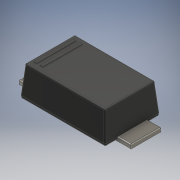
# Autodesk Inventor part: Semiconductor_DO219AB
Saved by Autodesk Inventor 2018 (Build 220112000, 112)
## iProperties
Created: 2018-09-29
Part Number: Semiconductor_DO219AB
Material: ABS Plastic
Document SubType Name: Modeling
Designer: Bradley
Density: 1.06 g/cm^3
Appearance: Smooth - Black
Author: Bradley
Autodesk Inventor part; units mm, degrees
ref_plane "YZ Plane" through (0, 0, 0) normal (1, 0, 0) x (0, 1, 0)
ref_plane "XZ Plane" through (0, 0, 0) normal (0, 1, 0) x (-1, 0, 0)
ref_plane "XY Plane" through (0, 0, 0) normal (0, 0, 1) x (1, 0, 0)
sketch "Sketch1" plane through (0, 0, 0) normal (0, 0, 1) x (1, 0, 0)
  line L0 (-1.4, -0.9) -> (1.4, -0.9)
  line L1 (1.4, -0.9) -> (1.4, 0.9)
  line L2 (1.4, 0.9) -> (-1.4, 0.9)
  line L3 (-1.4, 0.9) -> (-1.4, -0.9)
  line L4 (-1.4, -0.9) -> (1.4, 0.9) construction
  line L5 (1.4, -0.9) -> (-1.4, 0.9) construction
  point P0 (0, 0)
  dimension "d0" = 2.8
  dimension "d1" = 1.8
  constraints: 12 end point, 2 midpoint, 2 parallel, 1 horizontal, 1 perpendicular
  measures "d0" distance of L2.end L1.end
  measures "d1" distance of L1.end L0.end
extrude "Extrusion1" add sketch "Sketch1" along normal blind 0.9 draft -5 and the other way blind 0.1 draft -5
sketch "Sketch2" plane through (0, 0, 0) normal (0, 0, 1) x (1, 0, 0)
  line L0 (-1.3213, -0.8213) -> (-1.3213, 0.8213) projected
  line L1 (-1.4, 0.9) -> (-1.3213, 0.8213) projected
  line L2 (-1.4, 0.9) -> (-1.4, -0.9) projected
  line L3 (-1.4, -0.9) -> (-1.3213, -0.8213) projected
  line L4 (-1.3213, 0.8213) -> (1.3213, 0.8213) projected
  line L5 (1.4, 0.9) -> (1.3213, 0.8213) projected
  line L6 (1.4, 0.9) -> (-1.4, 0.9) projected
  line L7 (-1.4, 0.9) -> (-1.3213, 0.8213) projected
  line L8 (1.3213, 0.8213) -> (1.3213, -0.8213) projected
  line L9 (1.4, -0.9) -> (1.3213, -0.8213) projected
  line L10 (1.4, -0.9) -> (1.4, 0.9) projected
  line L11 (1.4, 0.9) -> (1.3213, 0.8213) projected
  line L12 (1.3213, -0.8213) -> (-1.3213, -0.8213) projected
  line L13 (-1.4, -0.9) -> (-1.3213, -0.8213) projected
  line L14 (-1.4, -0.9) -> (1.4, -0.9) projected
  line L15 (1.4, -0.9) -> (1.3213, -0.8213) projected
  line L16 (-1.85, 0.5) -> (-1.25, 0.5)
  line L17 (-1.25, 0.5) -> (-1.25, -0.5)
  line L18 (-1.25, -0.5) -> (-1.85, -0.5)
  line L19 (-1.85, -0.5) -> (-1.85, 0.5)
  line L20 (1.85, 0.5) -> (1.25, 0.5)
  line L21 (1.25, 0.5) -> (1.25, -0.5)
  line L22 (1.25, -0.5) -> (1.85, -0.5)
  line L23 (1.85, -0.5) -> (1.85, 0.5)
  line L24 (-1.85, 0) -> (1.85, 0) construction
  point P0 (0, 0)
  point P1 (0, 0)
  dimension "d6" = 1
  dimension "d7" = 3.7
  dimension "d8" = 0.6
  constraints: 18 end point, 4 parallel, 3 collinear, 3 midpoint, 2 horizontal, 2 perpendicular, 1 coincident
  measures "d6" distance of L18.end L16.start
  measures "d7" distance between parallel lines of L23 L19
  measures "d8" distance of L16.start L16.end
extrude "Extrusion2" add sketch "Sketch2" against normal blind 0.15 contours L18 L2 L16 L0 | L0 L16 L17 L18 | L18 L19 L16 L2 | L22 L21 L20 L8 | L8 L20 L10 L22 | L10 L20 L23 L22
sketch "Sketch3" plane through (0, 0, 0.9) normal (0, 0, 1) x (1, 0, 0)
  line L0 (-1.2, 0.65) -> (-1.1, 0.65)
  line L1 (-1.1, 0.65) -> (-1.1, -0.65)
  line L2 (-1.1, -0.65) -> (-1.2, -0.65)
  line L3 (-1.2, -0.65) -> (-1.2, 0.65)
  line L4 (-1, 0.65) -> (-0.9, 0.65)
  line L5 (-0.9, 0.65) -> (-0.9, -0.65)
  line L6 (-0.9, -0.65) -> (-1, -0.65)
  line L7 (-1, -0.65) -> (-1, 0.65)
  point P0 (0, 0)
  point P1 (-0.9, 0)
  dimension "d11" = 0.1
  dimension "d12" = 0.1
  dimension "d13" = 1.3
  dimension "d14" = 0.9
  constraints: 16 end point, 4 parallel, 2 horizontal, 2 perpendicular, 2 point on line, 1 collinear, 1 horizontal alignment, 1 midpoint
  measures "d11" distance of L4.start L4.end
  measures "d12" distance between parallel lines of L7 L1
  measures "d13" distance of L4.end L5.end
  measures "d14" distance from line of L5 point (0, 0)
extrude "Extrusion3" add sketch "Sketch3" along normal blind 0.02
fillet "Fillet1" radius 0.05 18 edges at (-1.3606, -0.8606, 0.45) (-1.3956, -0.8956, -0.05) (-1.3213, 0, 0.9) (0, -0.8213, 0.9) (0, 0.8213, 0.9) (-1.3606, 0.8606, 0.45) (-1.3956, 0.8956, -0.05) (-1.3913, 0.6956, -0.1) (0, 0.8913, -0.1) (-1.3913, -0.6956, -0.1) (0, -0.8913, -0.1) (1.3956, -0.8956, -0.05) (1.3913, -0.6956, -0.1) (1.3606, -0.8606, 0.45) (1.3213, 0, 0.9) (1.3913, 0.6956, -0.1) (1.3956, 0.8956, -0.05) (1.3606, 0.8606, 0.45)
fillet "Fillet2" radius 0.03 18 edges at (1.625, 0.5, 0) (1.85, 0, 0) (1.625, -0.5, 0) (1.85, -0.5, -0.075) (1.85, 0, -0.15) (1.55, 0.5, -0.15) (1.85, 0.5, -0.075) (1.25, 0, -0.15) (1.55, -0.5, -0.15) (-1.85, 0, -0.15) (-1.55, -0.5, -0.15) (-1.85, -0.5, -0.075) (-1.625, -0.5, 0) (-1.85, 0, 0) (-1.55, 0.5, -0.15) (-1.85, 0.5, -0.075) (-1.25, 0, -0.15) (-1.625, 0.5, 0)
equation "\"d12\" = d11"
body "Solid1"
